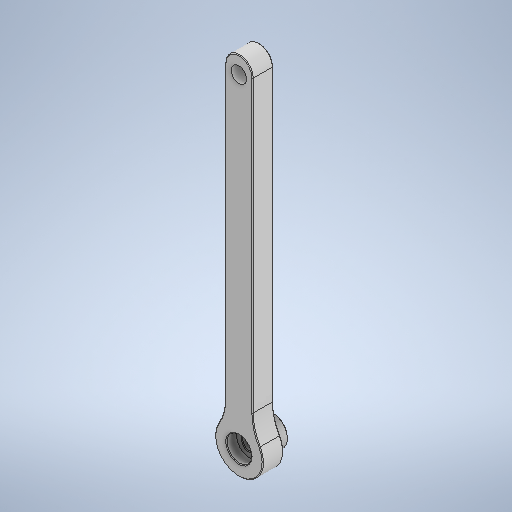
# Autodesk Inventor part: alternativeJoint
Saved by Autodesk Inventor 2025.1 (Build 291241000, 241)
## iProperties
Created: 2024-11-06
Part Number: alternativeJoint
Material: Generisch
Document SubType Name: Modeling
Designer: ZOMBULLI
Density: 1 g/cm^3
Appearance: Vorgabe
Author: ZOMBULLI
Autodesk Inventor part; units mm, degrees
ref_plane "YZ Plane" through (0, 0, 0) normal (1, 0, 0) x (0, 1, 0)
ref_plane "XZ Plane" through (0, 0, 0) normal (0, 1, 0) x (-1, 0, 0)
ref_plane "XY Plane" through (0, 0, 0) normal (0, 0, 1) x (1, 0, 0)
sketch "Skizze1" plane through (0, 0, 0) normal (0, 1, 0) x (-1, 0, 0)
  line L0 (0, 100) -> (0, 100)
  line L1 (-4, 96) -> (-4, 11.0905)
  line L2 (4, 11.0905) -> (4, 96)
  arc A0 (-6.0455, 3.5288) -> (6.0455, 3.5288) centre (0, 0) ccw
  arc A1 (4, 11.0905) -> (6.0455, 3.5288) centre (19, 11.0905) ccw
  arc A2 (-6.0455, 3.5288) -> (-4, 11.0905) centre (-19, 11.0905) ccw
  line L3 (0, -28.5657) -> (0, 122.3941) projected
  circle A3 centre (0, 95) radius 2.25
  arc A4 (0, 100) -> (-4, 96) centre (0, 96) ccw
  arc A5 (4, 96) -> (0, 100) centre (0, 96) ccw
  point P0 (0, 0)
  point P1 (4, 100)
  point P2 (-4, 5.7446)
  point P3 (-4, 100)
  point P4 (4, 5.7446)
  point P5 (0, 100)
  dimension "d2" = 14
  dimension "d4" = 15
  dimension "d5" = 15
  dimension "d10" = 0
  dimension "d11" = 100
  dimension "d33" = 4
  dimension "d34" = 4
  dimension "d49" = 95
  dimension "d50" = 4
  dimension "d51" = 4.5
  constraints: 12 point on circle, 8 tangent, 7 point on line, 6 centre point, 6 end point, 1 concentric, 1 horizontal, 1 parallel, 1 perpendicular
  measures "d2" diameter of A0
  measures "d4" radius of A1
  measures "d5" radius of A2
  measures "d10" distance of A0.centre point (0, 0)
  measures "d11" distance from line of point (0, 0) L0
  measures "d33" distance between parallel lines of L3 L1
  measures "d34" distance between parallel lines of L2 L3
  measures "d49" distance of point (0, 0) A3.centre
  measures "d50" radius of A4
  measures "d51" diameter of A3
extrude "Extrusion1" add sketch "Skizze1" along normal blind 6
sketch "Skizze8" plane through (0, 6, 0) normal (0, 1, 0) x (1, 0, 0)
  circle A0 centre (0, 0) radius 4.4
  dimension "d36" = 8.8
  constraints: 1 centre point, 1 coincident
  measures "d36" diameter of A0
extrude "Extrusion5" add sketch "Skizze8" along normal blind 4
fillet "Rundung3" radius 0.2 1 edges at (-4.4, 10, 0)
fillet "Rundung4" radius 0.2 10 edges at (-4.5204, 6, 7.1738) (-4, 6, 53.5453) (4, 6, 53.5453) (4.5204, 6, 7.1738) (0, 6, -7) (-4.5204, 0, 7.1738) (-4, 0, 53.5453) (4, 0, 53.5453) (4.5204, 0, 7.1738) (0, 0, -7)
sketch "Skizze10" plane through (0, 0, 0) normal (0, -1, 0) x (1, 0, 0)
  circle A0 centre (0, 0) radius 3.65
  dimension "d41" = 7.3
  constraints: 1 centre point, 1 coincident
  measures "d41" diameter of A0
extrude "Extrusion6" cut sketch "Skizze10" against normal blind 3
sketch "Skizze11" plane through (0, 3, 0) normal (0, -1, 0) x (1, 0, 0)
  circle A0 centre (0, 0) radius 2.1
  dimension "d44" = 4.2
  constraints: 1 centre point, 1 coincident
  measures "d44" diameter of A0
extrude "Extrusion7" cut sketch "Skizze11" against normal up to next
fillet "Rundung5" radius 0.2 2 edges at (-2.1, 3, 0) (-3.65, 0, 0)
fillet "Rundung6" radius 0.2 1 edges at (-2.1, 10, 0)
extrude "Extrusion8" cut sketch "Skizze1" along normal blind 10 contours A3 L3 | L3 A3
